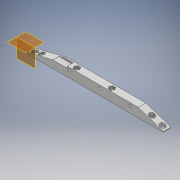
# Autodesk Inventor part: wheel_support_v4_narrow_with_line_sensor_all_holes
Saved by Autodesk Inventor 2018.2 (Build 222227000, 227)
## iProperties
Created: 2017-08-21
Part Number: wheel_support_v4_narrow_with_line_sensor_all_holes
Material: Generic
Document SubType Name: Modeling
Designer: ndz
Density: 1 g/cm^3
Appearance: Default
d1: 9,000 mm
d4: 3,200 mm
d6: 3,200 mm
d7: 3,200 mm
d8: 42,000 mm
d9: 60,500 mm
d13: 3,200 mm
d15: 3,200 mm
d17: 3,200 mm
d18: 36,500 mm
d26: 3,200 mm
d27: 48,000 mm
d28: 3,200 mm
d29: 42,000 mm
d32: 15,000 mm
d33: 5,000 mm
d39: 0,00 deg
d61: 3,200 mm
d62: 8,000 mm
d63: 12,500 mm
d64: 52,000 mm
d65: 36,500 mm
d67: 11,000 mm
d68: 0,00 deg
d70: 7,500 mm
d71: 0,00 deg
d78: 0,00 deg
d80: 10,000 mm
d81: 30,000 mm
d82: 3,000 mm
d83: 0,00 deg
d84: 8,500 mm
d85: 0,00 deg
d86: 10,000 mm
d87: 40,000 mm
d89: 0,00 deg
d92: 0,00 deg
d93: 5,900 mm
d94: 9,000 mm
d95: 0,00 deg
d97: 0,00 deg
d98: 5,900 mm
d99: 5,900 mm
d100: 5,900 mm
d102: 2,000 mm
d103: 17,000 mm
d104: 2,500 mm
d105: 7,300 mm
d106: 0,00 deg
d108: 4,000 mm
d109: 4,000 mm
d110: 4,000 mm
d111: 4,000 mm
d112: 4,000 mm
d114: 8,000 mm
d115: 73,000 mm
d2: 90,00 deg
d113: 4,000 mm
Author: ndz
Autodesk Inventor part; units mm, degrees
ref_plane "YZ Plane" through (0, 0, 0) normal (1, 0, 0) x (0, 1, 0)
ref_plane "XZ Plane" through (0, 0, 0) normal (0, 1, 0) x (-1, 0, 0)
ref_plane "XY Plane" through (0, 0, 0) normal (0, 0, 1) x (1, 0, 0)
sketch "Sketch1" plane through (0, 0, 0) normal (0, 0, 1) x (1, 0, 0)
  line L0 (0, 0) -> (164.5, 0)
  line L1 (164.5, 0) -> (164.5, 9)
  line L2 (164.5, 9) -> (0, 9)
  line L3 (0, 9) -> (0, 0)
  circle A0 centre (57, 4) radius 1.6
  circle A1 centre (99, 4) radius 1.6
  circle A2 centre (159.5, 4) radius 1.6
  circle A3 centre (147, 4) radius 1.6
  circle A4 centre (15, 4) radius 1.6
  circle A5 centre (7, 4) radius 1.6
  dimension "d1" = 9
  dimension "d2" = 90
  dimension "d4" = 3.2
  dimension "d6" = 3.2
  dimension "d7" = 3.2
  dimension "d8" = 42
  dimension "d9" = 60.5
  dimension "d26" = 3.2
  dimension "d27" = 48
  dimension "d28" = 3.2
  dimension "d29" = 42
  dimension "d32" = 15
  dimension "d33" = 5
  dimension "d61" = 3.2
  dimension "d62" = 8
  dimension "d63" = 12.5
  dimension "d108" = 4
  dimension "d109" = 4
  dimension "d110" = 4
  dimension "d111" = 4
  dimension "d112" = 4
  dimension "d113" = 4
  constraints: 8 end point, 6 centre point, 2 perpendicular, 1 horizontal
  measures "d1" distance of L0.end L1.end
  measures "d2" angle of L1 L0
  measures "d4" diameter of A0
  measures "d6" diameter of A1
  measures "d7" diameter of A2
  measures "d8" distance of A1.centre A0.centre
  measures "d9" distance of A2.centre A1.centre
  measures "d26" diameter of A3
  measures "d27" distance of A3.centre A1.centre
  measures "d28" diameter of A4
  measures "d29" distance of A4.centre A0.centre
  measures "d32" distance from line of L3 A4.centre
  measures "d33" distance from line of L1 A2.centre
  measures "d61" diameter of A5
  measures "d62" distance of A5.centre A4.centre
  measures "d63" distance of A2.centre A3.centre
  measures "d108" distance from line of L0 A5.centre
  measures "d109" distance from line of L0 A4.centre
  measures "d110" distance from line of L0 A0.centre
  measures "d111" distance from line of L0 A1.centre
  measures "d112" distance from line of L0 A3.centre
  measures "d113" distance from line of L0 A2.centre
ref_plane "Work Plane2" through (0, 0, 0) normal (0, -1, 0) x (1, 0, 0)
sketch "Sketch2" plane through (0, 0, 0) normal (0, -1, 0) x (1, 0, 0)
  circle A0 centre (52, 8) radius 1.6
  circle A1 centre (125, 8) radius 1.6
  circle A2 centre (88.5, 8) radius 1.6
  point P0 (0, 0)
  point P1 (52, 0)
  dimension "d13" = 3.2
  dimension "d15" = 3.2
  dimension "d17" = 3.2
  dimension "d18" = 36.5
  dimension "d64" = 52
  dimension "d65" = 36.5
  dimension "d114" = 8
  dimension "d115" = 73
  constraints: 3 centre point, 1 horizontal alignment, 2 other
  measures "d13" diameter of A0
  measures "d15" diameter of A1
  measures "d17" diameter of A2
  measures "d18" distance of A0.centre A2.centre
  measures "d64" horizontal distance of point (0, 0) A0.centre
  measures "d65" distance of A1.centre A2.centre
  measures "d114" distance of point (52, 0) A0.centre
  measures "d115" distance of A1.centre A0.centre
ref_plane "Work Plane1" through (0, 0, 11) normal (0, 0, 1) x (1, 0, 0)
extrude "klocek" add sketch "Sketch1" along normal blind 11
ref_plane "Work Plane3" through (0, 0, 0) normal (0, -1, 0) x (1, 0, 0)
extrude "prowadzenie osi" cut sketch "Sketch2" against normal up to next
ref_plane "Work Plane4" through (0, 0, 0) normal (0, -1, 0) x (1, 0, 0)
sketch "Sketch7" plane through (0, 0, 0) normal (0, -1, 0) x (1, 0, 0)
  line L0 (0, 11) -> (0, 1)
  line L1 (0, 11) -> (164.5, 11) projected
  line L2 (0, 11) -> (40, 11)
  line L3 (40, 11) -> (0, 1)
  point P0 (0, -1.8333)
  dimension "d86" = 10
  dimension "d87" = 40
  constraints: 6 end point, 1 point on line
  measures "d86" distance of L0.start L0.end
  measures "d87" distance of L0.start L2.end
sketch "Sketch8" plane through (0, 0, 0) normal (0, -1, 0) x (1, 0, 0)
  line L0 (164.5, 0) -> (164.5, 11) projected
  line L1 (164.5, 11) -> (164.5, 1)
  line L2 (164.5, 11) -> (0, 11) projected
  line L3 (164.5, 11) -> (134.5, 11)
  line L4 (134.5, 11) -> (164.5, 1)
  point P0 (0, 0)
  point P1 (40.8333, 11)
  dimension "d80" = 10
  dimension "d81" = 30
  constraints: 6 end point, 2 point on line
  measures "d80" distance of L0.end L1.end
  measures "d81" distance of L0.end L3.end
extrude "przedni skos" cut sketch "Sketch7" against normal up to next
extrude "tylni skos" cut sketch "Sketch8" against normal up to next
ref_plane "Work Plane7" through (0, 0, 11) normal (0, 0, 1) x (1, 0, 0)
sketch "Sketch5" plane through (0, 0, 11) normal (0, 0, 1) x (1, 0, 0)
  circle A0 centre (99, 4) radius 1.6 projected
  line L0 (95.5936, 4) -> (97.2968, 6.95)
  line L1 (97.2968, 6.95) -> (100.7032, 6.95)
  line L2 (100.7032, 6.95) -> (102.4064, 4)
  line L3 (102.4064, 4) -> (100.7032, 1.05)
  line L4 (100.7032, 1.05) -> (97.2968, 1.05)
  line L5 (97.2968, 1.05) -> (95.5936, 4)
  circle A1 centre (57, 4) radius 1.6 projected
  line L6 (60.4064, 4) -> (58.7032, 1.05)
  line L7 (58.7032, 1.05) -> (55.2968, 1.05)
  line L8 (55.2968, 1.05) -> (53.5936, 4)
  line L9 (53.5936, 4) -> (55.2968, 6.95)
  line L10 (55.2968, 6.95) -> (58.7032, 6.95)
  line L11 (58.7032, 6.95) -> (60.4064, 4)
  point P0 (119.5, 5)
  dimension "d98" = 5.9
  dimension "d100" = 5.9
  constraints: 24 end point, 2 coincident, 26 other
  measures "d98" distance between parallel lines of L1 L4
  measures "d100" distance between parallel lines of L10 L7
extrude "hex insert middle" cut sketch "Sketch5" against normal blind 3
ref_plane "Work Plane6" through (0, 0, 11) normal (0, 0, 1) x (1, 0, 0)
sketch "Sketch9" plane through (0, 0, 11) normal (0, 0, 1) x (1, 0, 0)
  circle A0 centre (147, 4) radius 1.6 projected
  line L0 (150.4064, 4) -> (148.7032, 1.05)
  line L1 (148.7032, 1.05) -> (145.2968, 1.05)
  line L2 (145.2968, 1.05) -> (143.5936, 4)
  line L3 (143.5936, 4) -> (145.2968, 6.95)
  line L4 (145.2968, 6.95) -> (148.7032, 6.95)
  line L5 (148.7032, 6.95) -> (150.4064, 4)
  point P0 (0, 0)
  point P1 (153, 5)
  dimension "d99" = 5.9
  constraints: 12 end point, 1 coincident, 13 other
  measures "d99" distance between parallel lines of L4 L1
extrude "hex insert rear 1" cut sketch "Sketch9" against normal blind 7.5
ref_plane "Work Plane5" through (0, 0, 11) normal (0, 0, 1) x (1, 0, 0)
sketch "Sketch10" plane through (0, 0, 11) normal (0, 0, 1) x (1, 0, 0)
  circle A0 centre (159.5, 4) radius 1.6 projected
  line L0 (162.45, 5.7032) -> (162.45, 2.2968)
  line L1 (162.45, 2.2968) -> (159.5, 0.5936)
  line L2 (159.5, 0.5936) -> (156.55, 2.2968)
  line L3 (156.55, 2.2968) -> (156.55, 5.7032)
  line L4 (156.55, 5.7032) -> (159.5, 7.4064)
  line L5 (159.5, 7.4064) -> (162.45, 5.7032)
  line L6 (164.5, 0) -> (134.5, 0) projected
  point P0 (0, 0)
  dimension "d118" = 5.9
  constraints: 12 end point, 1 coincident, 1 perpendicular, 13 other
  measures "d118" distance between parallel lines of L1 L4
extrude "hex insert rear 2" cut sketch "Sketch10" against normal up to next contours A0 | L0 L1 L2 L3 L4 L5
sketch "Sketch13" plane through (0, 0, 11) normal (0, 0, 1) x (1, 0, 0)
  circle A0 centre (7, 4) radius 1.6 projected
  line L0 (10.4064, 4) -> (8.7032, 1.05)
  line L1 (8.7032, 1.05) -> (5.2968, 1.05)
  line L2 (5.2968, 1.05) -> (3.5936, 4)
  line L3 (3.5936, 4) -> (5.2968, 6.95)
  line L4 (5.2968, 6.95) -> (8.7032, 6.95)
  line L5 (8.7032, 6.95) -> (10.4064, 4)
  dimension "d123" = 5.9
  constraints: 12 end point, 1 coincident, 13 other
  measures "d123" distance between parallel lines of L0 L3
extrude "hex insert front 1" cut sketch "Sketch13" against normal through all
sketch "Sketch16" plane through (0, 0, 11) normal (0, 0, 1) x (1, 0, 0)
  circle A0 centre (15, 4) radius 1.6 projected
  line L0 (18.4064, 4) -> (16.7032, 1.05)
  line L1 (16.7032, 1.05) -> (13.2968, 1.05)
  line L2 (13.2968, 1.05) -> (11.5936, 4)
  line L3 (11.5936, 4) -> (13.2968, 6.95)
  line L4 (13.2968, 6.95) -> (16.7032, 6.95)
  line L5 (16.7032, 6.95) -> (18.4064, 4)
  point P0 (0, 0)
  dimension "d93" = 5.9
  constraints: 12 end point, 1 coincident, 13 other
  measures "d93" distance between parallel lines of L1 L4
extrude "hex insert front 2" cut sketch "Sketch16" against normal blind 9
sketch "Sketch17" plane through (0, 0, 0) normal (0, 0, -1) x (-1, 0, 0)
  line L0 (-164.5, 9) -> (0, 9) projected
  line L1 (0, 0) -> (-2, 0)
  line L2 (-2, 0) -> (-2, 9)
  line L3 (-2, 9) -> (0, 9)
  line L4 (0, 9) -> (0, 0)
  dimension "d122" = 2
  constraints: 8 end point, 2 parallel, 1 horizontal, 1 perpendicular, 1 point on line
  measures "d122" distance between parallel lines of L2 L4
extrude "ciecie przod" cut sketch "Sketch17" against normal up to next
sketch "Sketch18" plane through (40, 0, 11) normal (0, -1, 0) x (1, 0, 0)
  line L0 (9.5, 0) -> (9.5, -2)
  line L1 (9.5, -2) -> (-7.5, -2)
  line L2 (-7.5, -2) -> (-7.5, 0)
  line L3 (-7.5, 0) -> (9.5, 0)
  line L4 (94.5, 0) -> (0, 0) projected
  circle A0 centre (12, -3) radius 1.6 projected
  line L5 (-40, -11) -> (124.5, -11) projected
  point P0 (-35, -11)
  dimension "d102" = 2
  dimension "d103" = 17
  dimension "d104" = 2.5
  constraints: 8 end point, 2 collinear, 2 perpendicular, 1 parallel, 1 vertical
  measures "d102" distance of L0.start L0.end
  measures "d103" distance of L0.end L1.end
  measures "d104" distance from line of L0 A0.centre
extrude "sensor linii" cut sketch "Sketch18" against normal blind 7.3 contours L0 L1 L2 L3
body "Solid1"
